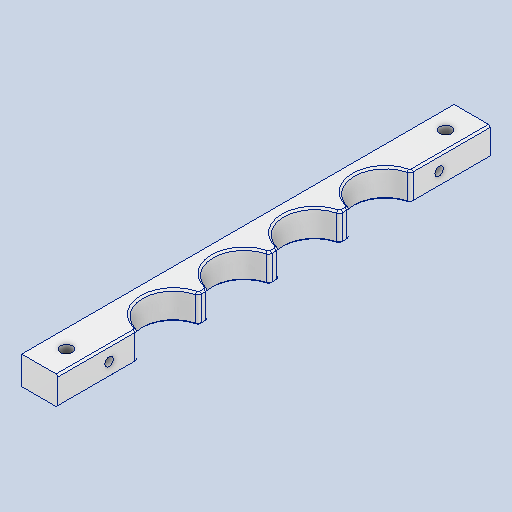
# Autodesk Inventor part: BatteryHolder
Saved by Autodesk Inventor 2023 (Build 270158000, 158)
## iProperties
Created: 2022-08-06
Part Number: BatteryHolder
Material: Aluminum 6061
Document SubType Name: Modeling
Designer: Aditya Bansal
Density: 2.7 g/cm^3
Appearance: Aluminum - Flat
Author: Aditya Bansal
Autodesk Inventor part; units mm, degrees
ref_plane "YZ Plane" through (0, 0, 0) normal (1, 0, 0) x (0, 1, 0)
ref_plane "XZ Plane" through (0, 0, 0) normal (0, 1, 0) x (-1, 0, 0)
ref_plane "XY Plane" through (0, 0, 0) normal (0, 0, 1) x (1, 0, 0)
sketch "Sketch1" plane through (0, 0, 0) normal (0, 1, 0) x (-1, 0, 0)
  line L0 (0, 0) -> (11.75, 0)
  line L1 (11.75, 0) -> (11.75, -107.5)
  line L2 (10.25, -107.5) -> (0, -107.5)
  line L3 (0, -107.5) -> (0, 0)
  circle A0 centre (11.75, -23.75) radius 8.75
  circle A1 centre (11.75, -43.75) radius 8.75
  circle A2 centre (11.75, -63.75) radius 8.75
  circle A3 centre (11.75, -83.75) radius 8.75
  line L4 (11.75, 0) -> (23.5, 0)
  line L5 (23.5, 0) -> (23.5, -107.5)
  line L6 (23.5, -107.5) -> (13.25, -107.5)
  line L7 (13.25, -107.5) -> (13.25, -92.3705)
  line L8 (13.25, -75.1295) -> (13.25, -72.3705)
  line L9 (13.25, -55.1295) -> (13.25, -52.3705)
  line L10 (13.25, -32.3705) -> (13.25, -35.1295)
  line L11 (13.25, -15.1295) -> (13.25, 0)
  line L12 (10.25, -52.3705) -> (10.25, -55.1295)
  line L13 (10.25, -107.5) -> (13.25, -107.5)
  line L14 (23.5, 0) -> (13.25, 0)
  line L15 (13.25, 0) -> (13.25, 7.5)
  line L16 (13.25, 7.5) -> (23.5, 7.5)
  line L17 (23.5, 7.5) -> (23.5, 0)
  line L18 (11.75, -107.5) -> (23.5, -107.5)
  line L19 (23.5, -107.5) -> (23.5, -115)
  line L20 (23.5, -115) -> (13.25, -115)
  line L21 (13.25, -115) -> (13.25, -107.5)
  point P0 (11.75, -92.5)
  point P1 (11.75, -75)
  point P2 (11.75, -72.5)
  point P3 (11.75, -55)
  point P4 (11.75, -52.5)
  point P5 (11.75, -35)
  point P6 (11.75, -32.5)
  point P7 (11.75, -15)
  point P8 (13.25, -99.9352)
  dimension "d0" = 17.5
  dimension "d4" = 20
  dimension "d9" = 3
  dimension "d11" = 15
  dimension "d12" = 15
  dimension "d16" = 1.5
  dimension "d17" = 3
  dimension "d57" = 7.5
  constraints: 44 end point, 10 point on circle, 8 collinear, 8 point on line, 7 perpendicular, 6 parallel, 5 horizontal, 4 centre point, 2 vertical, 1 midpoint, 6 other
  measures "d0" diameter of A0
  measures "d4" distance of A0.centre A1.centre
  measures "d9" distance edge to line of A3 L3
  measures "d11" distance edge to line of A3 L2
  measures "d12" distance edge to line of A0 L0
  measures "d16" distance between parallel lines of L1 L7
  measures "d17" distance edge to line of A3 L5
  measures "d57" distance between parallel lines of L20 L6
extrude "Extrusion1" add sketch "Sketch1" along normal blind 8 contours L15 L16 L17 L4 | L4 L5 L6 L7 A3 L8 A2 L9 A1 L10 A0 L11 | L19 L20 L21 L6
sketch "Sketch3" plane through (-23.5, 0, -100) normal (-1, 0, 0) x (0, 0, 1)
  line L0 (-15, 0) -> (-15, 8) projected
  line L1 (107.5, 0) -> (107.5, 8) projected
  point P0 (-0.5, 4)
  point P1 (93, 4)
  point P2 (107.5, 4)
  dimension "d42" = 14.5
  dimension "d43" = 14.5
  constraints: 2 horizontal alignment, 1 midpoint
  measures "d42" distance from line of point (-0.5, 4) L0
  measures "d43" distance of point (93, 4) point (107.5, 4)
hole "Hole1" at (-23.5, 4, -100.5) at (-23.5, 4, -7) direction (1, 0, 0) diameter 2.459 end through all thread size "M3x0.5" class "6H" standard "ANSI Metric M Profile"
sketch "Sketch4" plane through (0, 0, 0) normal (0, -1, 0) x (1, 0, 0)
  line L0 (-23.5, -115) -> (-23.5, 7.5) projected
  line L1 (-13.25, 7.5) -> (-13.25, -15.1295) projected
  line L2 (-13.25, -115) -> (-23.5, -115) projected
  line L3 (-23.5, 7.5) -> (-13.25, 7.5) projected
  point P0 (0, 0)
  point P1 (-18.375, 0)
  point P2 (-18.375, -107.5)
  point P3 (-18.375, -115)
  dimension "d51" = 10.25
  dimension "d52" = 5.125
  dimension "d53" = 7.5
  dimension "d54" = 7.5
  constraints: 1 midpoint, 1 vertical alignment
  measures "d51" distance between parallel lines of L0 L1
  measures "d52" distance from line of L0 point (-18.375, 0)
  measures "d53" distance of point (-18.375, -115) point (-18.375, -107.5)
  measures "d54" distance from line of point (-18.375, 0) L3
hole "Hole2" at (-18.375, 0, -107.5) at (-18.375, 0, 0) direction (0, 1, 0) diameter 3.4 end through all clearance for "Flat Head Machine Screw" size "M3" standard "Ansi Metric M Profile"
fillet "Fillet1" radius 1 8 edges at (-13.25, 4, -92.3705) (-13.25, 4, -72.3705) (-13.25, 4, -75.1295) (-13.25, 4, -55.1295) (-13.25, 4, -52.3705) (-13.25, 4, -35.1295) (-13.25, 4, -32.3705) (-13.25, 4, -15.1295)
chamfer "Chamfer1" distance 0.5 angle 45 30 edges at (-20.5, 0, -83.75) (-13.4574, 0, -92.5643) (-13.4574, 0, -74.9357) (-13.25, 0, -73.75) (-13.4574, 0, -72.5643) (-20.5, 0, -63.75) (-13.4574, 0, -54.9357) (-13.25, 0, -53.75) (-13.4574, 0, -52.5643) (-20.5, 0, -43.75) (-13.4574, 0, -34.9357) (-13.25, 0, -33.75) (-13.4574, 0, -32.5643) (-20.5, 0, -23.75) (-13.4574, 0, -14.9357) (-20.5, 8, -23.75) (-13.4574, 8, -32.5643) (-13.25, 8, -33.75) (-13.4574, 8, -34.9357) (-20.5, 8, -43.75) (-13.4574, 8, -52.5643) (-13.25, 8, -53.75) (-13.4574, 8, -54.9357) (-20.5, 8, -63.75) (-13.4574, 8, -72.5643) (-13.25, 8, -73.75) (-13.4574, 8, -74.9357) (-20.5, 8, -83.75) (-13.4574, 8, -92.5643) (-13.4574, 8, -14.9357)
equation "\"d12\" = d11"
equation "\"d43\" = d42"
equation "\"d52\" = 0.5 * d51"
equation "\"d54\" = d53"
body "Solid1"
